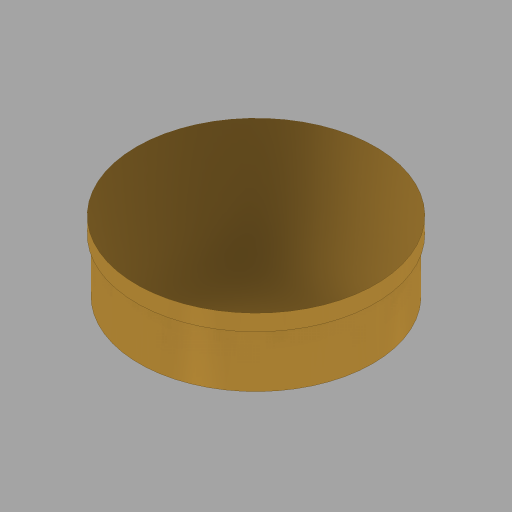
# Autodesk Inventor part: CapCenterThin
Saved by Autodesk Inventor 2024 (Build 280153020, 153B)
## iProperties
Created: 2023-09-22
Part Number: CapCenterThin
Material: Brass
Document SubType Name: Modeling
Designer: schanen
Density: 8.49 g/cm^3
Appearance: Brass - Polished
Author: schanen
Autodesk Inventor part; units mm, degrees
ref_plane "YZ Plane" through (0, 0, 0) normal (1, 0, 0) x (0, 1, 0)
ref_plane "XZ Plane" through (0, 0, 0) normal (0, 1, 0) x (-1, 0, 0)
ref_plane "XY Plane" through (0, 0, 0) normal (0, 0, 1) x (1, 0, 0)
sketch "Sketch1" plane through (0, 0, 0) normal (0, 0, 1) x (1, 0, 0)
  line L0 (-22.225, 13) -> (0, 13)
  line L1 (0, 13) -> (0, 10)
  line L2 (0, 10) -> (-20, 10)
  line L3 (-21.725, 0) -> (-20, 0)
  line L4 (-21.725, 0) -> (-21.725, 10)
  line L5 (-21.725, 10) -> (-22.225, 10)
  line L6 (-22.225, 10) -> (-22.225, 13)
  line L7 (-21.725, -10) -> (-22.225, -10) construction
  line L8 (-22.225, -10) -> (-22.225, 0) construction
  line L9 (-22.225, 0) -> (-21.725, 0) construction
  line L10 (-21.725, 0) -> (-21.725, -10) construction
  line L11 (-20, 10) -> (-20, 0)
  line L12 (-6, 10) -> (-8, 10)
  line L13 (-8, 10) -> (-8, 0)
  line L14 (-8, 0) -> (-6, 0)
  line L15 (-6, 0) -> (-6, 10)
  point P0 (0, 0)
  point P1 (-8, 10)
  dimension "d16" = 3
  dimension "d20" = 0.5
  dimension "d21" = 10
  dimension "d22" = 22.225
  dimension "d25" = 10
  dimension "d27" = 22.225
  dimension "d28" = 8
  dimension "d29" = 2
  dimension "d30" = 10
  dimension "d35" = 20
  constraints: 32 end point, 6 perpendicular, 4 horizontal, 4 horizontal alignment, 4 parallel, 2 vertical, 2 vertical alignment, 1 coincident, 1 point on line
  measures "d16" distance of L0.end L1.end
  measures "d20" distance of L8.end L9.end
  measures "d21" distance of L7.end L8.end
  measures "d22" distance from line of point (0, 0) L8
  measures "d25" distance of L3.start L4.end
  measures "d27" distance of L0.start L0.end
  measures "d28" distance from line of point (0, 0) L13
  measures "d29" distance between parallel lines of L13 L15
  measures "d30" distance from line of L2 L14.end
  measures "d35" distance from line of point (0, 0) L11
revolve "Revolution1" add sketch "Sketch1" angle 360 about axis through (0, 13, 0) along (0, -1, 0)
fillet "Fillet1" radius 1 1 edges at (6, 0, 0)
body "Solid1"
